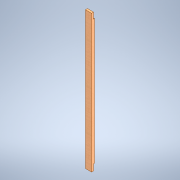
# Autodesk Inventor part: sidev2
Saved by Autodesk Inventor 2020 (Build 240168000, 168)
## iProperties
Created: 2020-05-19
Part Number: sidev2
Material: Wood (Cherry)
Document SubType Name: Modeling
Designer: kolbe
Density: 0.63 g/cm^3
Appearance: Cherry - Natural Low Gloss
Author: kolbe
Autodesk Inventor part; units mm, degrees
ref_plane "YZ Plane" through (0, 0, 0) normal (1, 0, 0) x (0, 1, 0)
ref_plane "XZ Plane" through (0, 0, 0) normal (0, 1, 0) x (-1, 0, 0)
ref_plane "XY Plane" through (0, 0, 0) normal (0, 0, 1) x (1, 0, 0)
sketch "Sketch1" plane through (0, 0, 0) normal (1, 0, 0) x (0, 1, 0)
  line L0 (0, 0) -> (863.6, 0)
  line L1 (863.6, 0) -> (863.6, -19.05)
  line L2 (863.6, -19.05) -> (0, -19.05)
  line L3 (0, -19.05) -> (0, 0)
  dimension "d0" = 863.6
  dimension "d1" = 19.05
  constraints: 8 end point, 2 parallel, 1 horizontal, 1 perpendicular
  measures "d0" distance of L1.end L2.end
  measures "d1" distance of L0.end L1.end
extrude "Extrusion1" add sketch "Sketch1" against normal blind 38.1
sketch "Sketch2" plane through (0, 0, 0) normal (1, 0, 0) x (0, 0, -1)
  line L0 (19.05, 0) -> (0, 0) projected
  line L1 (19.05, 0) -> (12.7, 0)
  line L2 (12.7, 0) -> (12.7, 38.1)
  line L3 (12.7, 38.1) -> (19.05, 38.1)
  line L4 (19.05, 38.1) -> (19.05, 0)
  point P0 (12.7, 0)
  dimension "d4" = 6.35
  dimension "d5" = 38.1
  constraints: 8 end point, 2 parallel, 1 horizontal, 1 perpendicular
  measures "d4" distance of L2.end L3.end
  measures "d5" distance of L1.end L2.end
extrude "Extrusion2" cut sketch "Sketch2" against normal blind 38.1
sketch "Sketch3" plane through (0, 0, 0) normal (1, 0, 0) x (0, 0, -1)
  line L0 (19.05, 38.1) -> (19.05, 863.6) projected
  line L1 (19.05, 863.6) -> (12.7, 863.6)
  line L2 (12.7, 863.6) -> (12.7, 825.5)
  line L3 (12.7, 825.5) -> (19.05, 825.5)
  line L4 (19.05, 825.5) -> (19.05, 863.6)
  point P0 (0, 0)
  dimension "d8" = 6.35
  dimension "d9" = 38.1
  constraints: 8 end point, 2 parallel, 1 horizontal, 1 perpendicular
  measures "d8" distance of L3.end L2.end
  measures "d9" distance of L2.end L1.end
extrude "Extrusion3" cut sketch "Sketch3" against normal blind 38.1
sketch "Sketch4" plane through (0, 38.1, -19.05) normal (0, 0, -1) x (-1, 0, 0)
  line L0 (38.1, 0) -> (38.1, -38.1) projected
  line L1 (38.1, 0) -> (31.75, 0)
  line L2 (31.75, 0) -> (31.75, 787.4)
  line L3 (31.75, 787.4) -> (38.1, 787.4)
  line L4 (38.1, 787.4) -> (38.1, 0)
  point P0 (0, -38.1)
  dimension "d12" = 6.35
  dimension "d13" = 787.4
  constraints: 8 end point, 2 parallel, 1 horizontal, 1 perpendicular
  measures "d12" distance of L2.end L3.end
  measures "d13" distance of L1.end L2.end
extrude "Extrusion4" cut sketch "Sketch4" against normal blind 9.525
body "Solid1"
